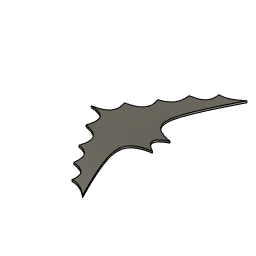
Bat (Autodesk Fusion 360 design; units mm, degrees)
Autodesk Fusion 360 part; units mm, degrees
sketch "Sketch1" plane through (0, 0, 0) normal (0, 0, 1) x (1, 0, 0)
  spline S0 degree 5 poles (20, 5) (19.6208, 4.8) (18.8954, 4.4) (17.9067, 3.8) (16.7905, 3) (15.7547, 2) (15.1106, 1) (14.89, 0) (15.1106, -1) (15.7547, -2) (16.7905, -3) (17.9067, -3.8) (18.8954, -4.4) (19.6208, -4.8) (20, -5) knots 0 0 0 0 0 0 0.1 0.2 0.3 0.4 0.5 0.6 0.7 0.8 0.9 1 1 1 1 1 1
  spline S1 degree 5 poles (20, 5) (19.2712, 5.1081) (17.8733, 5.3538) (15.9554, 5.8111) (13.759, 6.5997) (11.6261, 7.8912) (10.1129, 9.4979) (9.2114, 11.428) (8.8832, 13.6833) (9.0671, 16.2602) (9.6928, 19.1509) (10.6903, 22.3442) (11.9999, 25.8244) (13.5744, 29.5733) (15.3779, 33.5733) (17.3852, 37.8091) (19.1413, 41.3771) (20.5394, 44.1509) (21.5072, 46.0431) (22, 47) knots 0 0 0 0 0 0 0.066667 0.133333 0.2 0.266667 0.333333 0.4 0.466667 0.533333 0.6 0.666667 0.733333 0.8 0.866667 0.933333 1 1 1 1 1 1
  spline S2 degree 5 poles (20, -5) (19.2712, -5.1081) (17.8733, -5.3538) (15.9554, -5.8111) (13.759, -6.5997) (11.6261, -7.8912) (10.1129, -9.4979) (9.2114, -11.428) (8.8832, -13.6833) (9.0671, -16.2602) (9.6928, -19.1509) (10.6903, -22.3442) (11.9999, -25.8244) (13.5744, -29.5733) (15.3779, -33.5733) (17.3852, -37.8091) (19.1413, -41.3771) (20.5394, -44.1509) (21.5072, -46.0431) (22, -47) knots 0 0 0 0 0 0 0.066667 0.133333 0.2 0.266667 0.333333 0.4 0.466667 0.533333 0.6 0.666667 0.733333 0.8 0.866667 0.933333 1 1 1 1 1 1
  spline S3 degree 5 poles (22, 47) (21.7727, 46.8021) (21.3189, 46.4146) (20.6399, 45.8581) (19.7383, 45.1666) (18.6179, 44.3921) (17.5049, 43.7166) (16.4, 43.1495) (15.3036, 42.6985) (14.2158, 42.3629) (13.136, 42.1358) (12.2781, 42.0345) (11.6378, 42.001) (11.2124, 41.9972) (11, 42) knots 0 0 0 0 0 0 0.1 0.2 0.3 0.4 0.5 0.6 0.7 0.8 0.9 1 1 1 1 1 1
  spline S4 degree 5 poles (22, -47) (21.7727, -46.8021) (21.3189, -46.4146) (20.6399, -45.8581) (19.7383, -45.1666) (18.6179, -44.3921) (17.5049, -43.7166) (16.4, -43.1495) (15.3036, -42.6985) (14.2158, -42.3629) (13.136, -42.1358) (12.2781, -42.0345) (11.6378, -42.001) (11.2124, -41.9972) (11, -42) knots 0 0 0 0 0 0 0.1 0.2 0.3 0.4 0.5 0.6 0.7 0.8 0.9 1 1 1 1 1 1
  spline S5 degree 5 poles (11, 42) (11.0567, 41.6874) (11.1508, 41.074) (11.2338, 40.1895) (11.2264, 39.0824) (11.0075, 37.8268) (10.5616, 36.7102) (9.8726, 35.7422) (8.9361, 34.9257) (7.7664, 34.252) (6.3831, 33.7089) (5.1205, 33.3698) (4.0916, 33.1657) (3.3698, 33.0516) (3, 33) knots 0 0 0 0 0 0 0.1 0.2 0.3 0.4 0.5 0.6 0.7 0.8 0.9 1 1 1 1 1 1
  spline S6 degree 5 poles (11, -42) (11.0567, -41.6874) (11.1508, -41.074) (11.2338, -40.1895) (11.2264, -39.0824) (11.0075, -37.8268) (10.5616, -36.7102) (9.8726, -35.7422) (8.9361, -34.9257) (7.7664, -34.252) (6.3831, -33.7089) (5.1205, -33.3698) (4.0916, -33.1657) (3.3698, -33.0516) (3, -33) knots 0 0 0 0 0 0 0.1 0.2 0.3 0.4 0.5 0.6 0.7 0.8 0.9 1 1 1 1 1 1
  spline S7 degree 5 poles (3, 33) (3.0488, 32.6643) (3.1298, 32.003) (3.2017, 31.0414) (3.1969, 29.8211) (3.0117, 28.4056) (2.6312, 27.1097) (2.0398, 25.9431) (1.2292, 24.9109) (0.2085, 24.0075) (-1.0064, 23.2232) (-2.1209, 22.683) (-3.0317, 22.3239) (-3.6718, 22.1046) (-4, 22) knots 0 0 0 0 0 0 0.1 0.2 0.3 0.4 0.5 0.6 0.7 0.8 0.9 1 1 1 1 1 1
  spline S8 degree 5 poles (3, -33) (3.0519, -32.6532) (3.1391, -31.9722) (3.2199, -30.9891) (3.2258, -29.756) (3.0522, -28.3533) (2.6811, -27.1017) (2.0958, -26.0139) (1.2865, -25.0975) (0.261, -24.3466) (-0.965, -23.749) (-2.0931, -23.3837) (-3.0168, -23.1691) (-3.6666, -23.052) (-4, -23) knots 0 0 0 0 0 0 0.1 0.2 0.3 0.4 0.5 0.6 0.7 0.8 0.9 1 1 1 1 1 1
  spline S9 degree 5 poles (-4, 22) (-3.8671, 21.6411) (-3.6275, 20.9356) (-3.3469, 19.9148) (-3.1327, 18.6296) (-3.149, 17.1578) (-3.4725, 15.8318) (-4.1248, 14.6617) (-5.1107, 13.6499) (-6.4105, 12.787) (-7.9976, 12.0604) (-9.4768, 11.5784) (-10.6963, 11.2692) (-11.5574, 11.0859) (-12, 11) knots 0 0 0 0 0 0 0.1 0.2 0.3 0.4 0.5 0.6 0.7 0.8 0.9 1 1 1 1 1 1
  spline S10 degree 5 poles (-4, -23) (-3.8615, -22.5957) (-3.6109, -21.8015) (-3.3142, -20.6538) (-3.0793, -19.2121) (-3.0716, -17.5674) (-3.3744, -16.0936) (-4.0114, -14.8039) (-4.9925, -13.7036) (-6.3007, -12.7834) (-7.91, -12.029) (-9.4177, -11.5468) (-10.6645, -11.249) (-11.5464, -11.0783) (-12, -11) knots 0 0 0 0 0 0 0.1 0.2 0.3 0.4 0.5 0.6 0.7 0.8 0.9 1 1 1 1 1 1
  spline S11 degree 5 poles (-12, 11) (-11.8671, 10.6411) (-11.6275, 9.9356) (-11.3469, 8.9148) (-11.1327, 7.6296) (-11.149, 6.1578) (-11.4725, 4.8318) (-12.1248, 3.6617) (-13.1107, 2.6499) (-14.4105, 1.787) (-15.9976, 1.0604) (-17.4768, 0.5784) (-18.6963, 0.2692) (-19.5574, 0.0859) (-20, 0) knots 0 0 0 0 0 0 0.1 0.2 0.3 0.4 0.5 0.6 0.7 0.8 0.9 1 1 1 1 1 1
  spline S12 degree 5 poles (-12, -11) (-11.8595, -10.5833) (-11.605, -9.7673) (-11.3024, -8.5952) (-11.0601, -7.1378) (-11.0439, -5.5036) (-11.3393, -4.0734) (-11.9708, -2.8631) (-12.9501, -1.8804) (-14.2612, -1.1149) (-15.8784, -0.5497) (-17.3964, -0.2443) (-18.653, -0.0926) (-19.5424, -0.0252) (-20, 0) knots 0 0 0 0 0 0 0.1 0.2 0.3 0.4 0.5 0.6 0.7 0.8 0.9 1 1 1 1 1 1
  point P0 (15, 0)
  point P1 (10, 10)
  point P2 (10, 20)
  point P3 (10, -10)
  point P4 (10, -20)
  point P5 (16, 43)
  point P6 (16, -43)
  point P7 (10, 36)
  point P8 (10, -36)
  point P9 (2, 26)
  point P10 (2, -26)
  point P11 (-4, 15)
  point P12 (-4, -15)
  point P13 (-12, 4)
  point P14 (-12, -3)
extrude "Extrude1" add sketch "Sketch1" along normal blind 1
